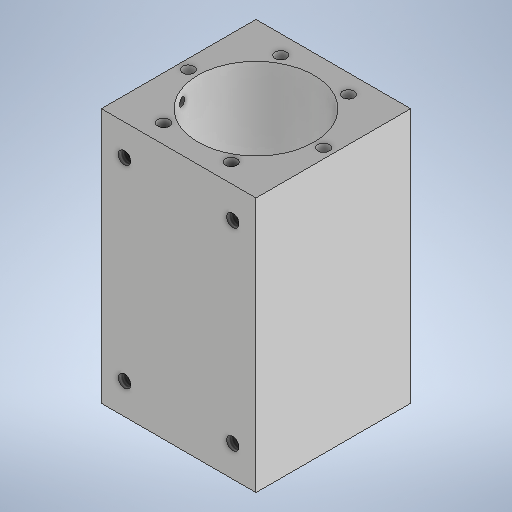
# Autodesk Inventor part: 06
Saved by Autodesk Inventor 2025.1 (Build 291241000, 241)
## iProperties
Created: 2024-09-13
Part Number: 06
Material: Generisch
Document SubType Name: Modeling
Designer: ffogue
Density: 1 g/cm^3
Appearance: Vorgabe
Author: ffogue
Autodesk Inventor part; units mm, degrees
ref_plane "YZ Plane" through (0, 0, 0) normal (1, 0, 0) x (0, 1, 0)
ref_plane "XZ Plane" through (0, 0, 0) normal (0, 1, 0) x (-1, 0, 0)
sketch "Sketch1" plane through (0, 0, 0) normal (0, 0, 1) x (1, 0, 0)
  line L0 (-20, -20) -> (20, -20)
  line L1 (20, -20) -> (20, 20)
  line L2 (20, 20) -> (-20, 20)
  line L3 (-20, 20) -> (-20, -20)
  line L4 (-20, -20) -> (20, 20) construction
  line L5 (20, -20) -> (-20, 20) construction
  point P0 (0, 0)
  dimension "d0" = 40
  dimension "d1" = 40
  constraints: 12 end point, 2 midpoint, 2 parallel, 1 horizontal, 1 perpendicular
  measures "d0" distance of L1.end L2.end
  measures "d1" distance of L2.end L0.start
extrude "Extrusion1" add sketch "Sketch1" along normal blind 66
sketch "Sketch2" plane through (0, 0, 66) normal (0, 0, 1) x (1, 0, 0)
  circle A0 centre (0, 0) radius 15
  circle A1 centre (0, 0) radius 17.5 construction
  line L0 (0, 0) -> (-8.75, 15.1554) construction
  line L1 (0, 0) -> (0, 15) construction
  circle A2 centre (-8.75, 15.1554) radius 1.5
  dimension "d4" = 30
  dimension "d5" = 35
  dimension "d61" = 30
  dimension "d62" = 3
  constraints: 4 end point, 3 coincident, 1 centre point, 1 vertical, 1 vertical alignment, 5 other
  measures "d61" angle of L1 L0
  measures "d62" diameter of A2
extrude "Extrusion2" cut sketch "Sketch2" against normal up to surface (66 mm away) contours A0
extrude "Extrusion3" cut sketch "Sketch2" against normal blind 10 contours A2
thread "Thread3" size "M3x0.5" class "6H" standard "ISO Metric profile" length 8
pattern_circular "Circular Pattern2" count 6 over 360 about axis through (0, 0, 66) along (0, 0, -1) of "Extrusion3"
sketch "Sketch3" plane through (-20, -20, 0) normal (-1, 0, 0) x (0, 0, 1)
  line L0 (17, 20) -> (49, 20) construction
  line L1 (17, 23) -> (49, 23)
  line L2 (49, 17) -> (17, 17)
  arc A0 (17, 23) -> (17, 17) centre (17, 20) ccw
  arc A1 (49, 17) -> (49, 23) centre (49, 20) ccw
  line L3 (0, 40) -> (66, 40) projected
  line L4 (0, 40) -> (0, 0) projected
  line L5 (31, 28) -> (35, 28) construction
  line L6 (31, 26) -> (35, 26)
  line L7 (35, 30) -> (31, 30)
  arc A2 (31, 30) -> (31, 26) centre (31, 28) ccw
  arc A3 (35, 26) -> (35, 30) centre (35, 28) ccw
  point P0 (0, 20)
  point P1 (33, 20)
  point P2 (33, 40)
  point P3 (0, 20)
  point P4 (33, 28)
  dimension "d19" = 3
  dimension "d20" = 32
  dimension "d21" = 2
  dimension "d22" = 4
  dimension "d23" = 8
  constraints: 16 end point, 8 point on circle, 8 tangent, 4 centre point, 4 midpoint, 2 horizontal, 2 parallel, 2 vertical alignment, 1 horizontal alignment
  measures "d19" radius of A0
  measures "d20" distance of L0.start L0.end
  measures "d21" radius of A2
  measures "d22" distance of L5.start L5.end
  measures "d23" distance between parallel lines of L0 L5
extrude "Extrusion4" cut sketch "Sketch3" against normal blind 3.5
sketch "Sketch4" plane through (-20, -20, 0) normal (-1, 0, 0) x (0, 0, 1)
  line L0 (0, 40) -> (66, 40) projected
  line L1 (0, 40) -> (0, 0) projected
  line L2 (0, 11) -> (66, 11) construction
  line L3 (66, 40) -> (66, 0) projected
  arc A0 (17, 23) -> (17, 17) centre (17, 20) ccw projected
  line L4 (0, 0) -> (66, 0) projected
  point P0 (0, 20)
  point P1 (42, 15)
  point P2 (42, 7)
  point P3 (24, 7)
  point P4 (24, 15)
  point P5 (33, 40)
  point P6 (14, 20)
  point P7 (3, 7)
  point P8 (63, 7)
  point P9 (3, 15)
  point P10 (63, 15)
  point P11 (33, 0)
  dimension "d28" = 8
  dimension "d29" = 9
  dimension "d30" = 30
  dimension "d31" = 60
  dimension "d32" = 18
  dimension "d33" = 9
  constraints: 6 horizontal alignment, 4 vertical alignment, 2 end point, 2 midpoint, 2 point on line, 1 horizontal, 1 point on circle, 1 symmetric about line
  measures "d28" distance of point (24, 7) point (24, 15)
  measures "d29" distance from line of L2 point (14, 20)
  measures "d30" horizontal distance of point (33, 40) point (3, 7)
  measures "d31" distance of point (63, 7) point (3, 7)
  measures "d32" distance of point (42, 7) point (24, 7)
  measures "d33" horizontal distance of point (33, 0) point (24, 7)
hole "Hole1" at (-20, -13, 3) at (-20, -13, 63) at (-20, -5, 3) at (-20, -5, 63) direction (1, 0, 0) diameter 2.013 depth 8 thread size "M2.5x0.45" class "6H" standard "ISO Metric profile"
hole "Hole2" at (-20, -5, 42) at (-20, -13, 42) at (-20, -13, 24) at (-20, -5, 24) direction (1, 0, 0) diameter 2.013 depth 8 thread size "M2.5x0.45" class "6H" standard "ISO Metric profile"
mirror "Mirror1" about plane through (0, 0, 0) normal (0, 1, 0) of "Hole2"
sketch "Sketch5" plane through (-20, -20, 0) normal (-1, 0, 0) x (0, 0, 1)
  line L0 (0, 11) -> (66, 11) construction
  circle A0 centre (3, 11) radius 2
  circle A1 centre (63, 11) radius 2
  line L1 (3, 9) -> (29, 9)
  line L2 (29, 9) -> (29, 10)
  line L3 (29, 10) -> (37, 10)
  line L4 (37, 10) -> (37, 9)
  line L5 (37, 9) -> (63, 9)
  line L6 (3, 13) -> (29, 13)
  line L7 (29, 13) -> (29, 14)
  line L8 (29, 14) -> (37, 14)
  line L9 (37, 14) -> (37, 13)
  line L10 (37, 13) -> (63, 13)
  circle A2 centre (24, 25) radius 1.0065 projected
  circle A3 centre (24, 33) radius 1.0065 projected
  circle A4 centre (42, 33) radius 1.0065 projected
  circle A5 centre (42, 25) radius 1.0065 projected
  circle A6 centre (24, 15) radius 1.0065 projected
  circle A7 centre (24, 7) radius 1.0065 projected
  circle A8 centre (42, 7) radius 1.0065 projected
  circle A9 centre (42, 15) radius 1.0065 projected
  circle A10 centre (63, 15) radius 1.0065 projected
  circle A11 centre (3, 15) radius 1.0065 projected
  circle A12 centre (63, 7) radius 1.0065 projected
  circle A13 centre (3, 7) radius 1.0065 projected
  line L11 (31, 30) -> (35, 30) projected
  arc A14 (35, 26) -> (35, 30) centre (35, 28) ccw projected
  line L12 (35, 26) -> (31, 26) projected
  arc A15 (31, 30) -> (31, 26) centre (31, 28) ccw projected
  arc A16 (17, 23) -> (17, 17) centre (17, 20) ccw projected
  line L13 (17, 23) -> (49, 23) projected
  arc A17 (49, 17) -> (49, 23) centre (49, 20) ccw projected
  line L14 (49, 17) -> (17, 17) projected
  line L15 (0, 40) -> (0, 0) projected
  line L16 (0, 0) -> (66, 0) projected
  line L17 (66, 40) -> (66, 0) projected
  line L18 (0, 40) -> (66, 40) projected
  point P0 (0, 20)
  point P1 (33, 10)
  point P2 (33, 14)
  point P3 (33, 0)
  dimension "d49" = 4
  dimension "d52" = 4
  dimension "d53" = 4
  dimension "d54" = 4
  dimension "d55" = 3
  dimension "d56" = 8
  constraints: 20 end point, 10 point on line, 4 perpendicular, 4 point on circle, 4 vertical alignment, 3 midpoint, 2 centre point, 2 tangent, 1 horizontal, 1 horizontal alignment, 1 parallel
  measures "d49" diameter of A1
  measures "d52" distance between parallel lines of L3 L8
  measures "d53" distance between parallel lines of L5 L10
  measures "d54" distance from line of point (33, 10) L8
  measures "d55" distance between parallel lines of L14 L8
  measures "d56" distance of L7.end L8.end
extrude "Extrusion5" cut sketch "Sketch5" against normal blind 4.5 contours A0 | A0 L6 L7 L8 L9 L10 A1 L5 L4 L3 L2 L1 | A1
fillet "Fillet1" radius 1 2 edges at (-17.75, -6, 29) (-17.75, -6, 37)
fillet "Fillet2" radius 1 2 edges at (-17.75, -10, 29) (-17.75, -10, 37)
sketch "Sketch6" plane through (-20, 20, 0) normal (0, 1, 0) x (1, 0, 0)
  line L0 (5, -3.5) -> (35, -3.5) construction
  line L1 (35, -3.5) -> (35, -62.5) construction
  line L2 (35, -62.5) -> (5, -62.5) construction
  line L3 (5, -62.5) -> (5, -3.5) construction
  line L4 (5, -3.5) -> (35, -62.5) construction
  line L5 (35, -3.5) -> (5, -62.5) construction
  line L6 (40, 0) -> (40, -66) projected
  line L7 (40, 0) -> (0, 0) projected
  point P0 (20, 0)
  point P1 (20, -33)
  point P2 (35, -33)
  point P3 (40, -33)
  point P4 (40, -33)
  point P5 (20, 0)
  dimension "d70" = 29.5
  dimension "d71" = 59
  dimension "d72" = 15
  dimension "d73" = 30
  constraints: 12 end point, 6 midpoint, 4 coincident, 2 parallel, 1 horizontal, 1 horizontal alignment, 1 perpendicular
  measures "d70" vertical distance of L0.end point (40, -33)
  measures "d71" distance of L0.end L1.end
  measures "d72" horizontal distance of point (20, 0) L0.end
  measures "d73" distance of L0.start L0.end
hole "Hole3" at (15, 20, 3.5) at (-15, 20, 3.5) at (-15, 20, 62.5) at (15, 20, 62.5) direction (0, -1, 0) diameter 2.459 depth 8.8 thread size "M3x0.5" class "6H" standard "ISO Metric profile"
sketch "Sketch7" plane through (-20, 20, 0) normal (0, 1, 0) x (1, 0, 0)
  line L0 (40, 0) -> (40, -66) projected
  line L1 (40, 0) -> (0, 0) projected
  point P0 (20, 0)
  point P1 (28, -33)
  point P2 (12, -33)
  point P3 (40, -33)
  point P4 (20, 0)
  dimension "d88" = 16
  dimension "d89" = 8
  constraints: 2 horizontal alignment, 2 midpoint
  measures "d88" distance of point (12, -33) point (28, -33)
  measures "d89" horizontal distance of point (20, 0) point (28, -33)
hole "Hole4" at (8, 20, 33) at (-8, 20, 33) direction (0, -1, 0) diameter 2.013 depth 5 thread size "M2.5x0.45" class "6H" standard "ISO Metric profile"
sketch "Sketch8" plane through (-20, -20, 0) normal (0, -1, 0) x (1, 0, 0)
  line L0 (34, 8) -> (6, 8) construction
  line L1 (6, 8) -> (6, 58) construction
  line L2 (6, 58) -> (34, 58) construction
  line L3 (34, 58) -> (34, 8) construction
  line L4 (34, 8) -> (6, 58) construction
  line L5 (6, 8) -> (34, 58) construction
  line L6 (0, 0) -> (40, 0) projected
  line L7 (0, 0) -> (0, 66) projected
  point P0 (20, 0)
  point P1 (20, 33)
  point P2 (20, 0)
  point P3 (6, 33)
  point P4 (0, 33)
  dimension "d90" = 50
  dimension "d91" = 28
  constraints: 12 end point, 5 midpoint, 4 coincident, 2 parallel, 1 horizontal, 1 horizontal alignment, 1 perpendicular, 1 vertical alignment
  measures "d90" distance of L0.end L1.end
  measures "d91" distance of L0.start L0.end
hole "Hole5" at (-14, -20, 8) at (14, -20, 8) at (-14, -20, 58) at (14, -20, 58) direction (0, 1, 0) diameter 3.242 depth 8 thread size "M4x0.7" class "6H" standard "ISO Metric profile"
ref_plane "Work Plane1" through (0, 0, 33) normal (0, 0, -1) x (-1, 0, 0)
mirror "Mirror2" about plane through (0, 0, 33) normal (0, 0, -1) of "Extrusion3", "Circular Pattern2"
equation "\"d49\" = d48"
equation "\"d73\" = 2 * d72"
equation "\"d89\" = 0.5 * d88"
equation "\"d48\" = 4"
body "Solid1"
